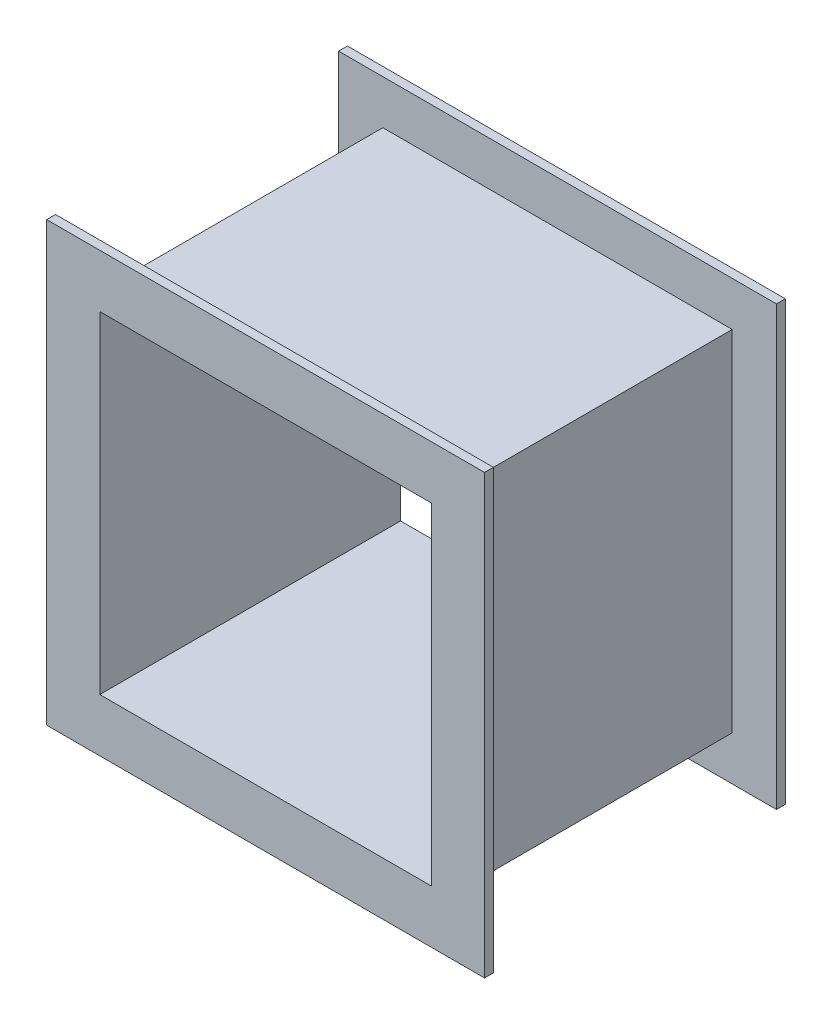
# Autodesk Inventor part: Измельчитель комков
Saved by Autodesk Inventor 2025 (Build 290162010, 162A)
## iProperties
Created: 2024-10-30
Part Number: Измельчитель комков
Material: Generic
Document SubType Name: Modeling
Designer: pokla
Density: 1 g/cm^3
Appearance: Default
Author: pokla
Autodesk Inventor part; units mm, degrees
ref_plane "YZ Plane" through (0, 0, 0) normal (1, 0, 0) x (0, 1, 0)
ref_plane "XZ Plane" through (0, 0, 0) normal (0, 1, 0) x (-1, 0, 0)
ref_plane "XY Plane" through (0, 0, 0) normal (0, 0, 1) x (1, 0, 0)
sketch "Sketch1" plane through (0, 0, 0) normal (0, 0, 1) x (1, 0, 0)
  line L0 (-247.5, 247.5) -> (247.5, 247.5)
  line L1 (247.5, 247.5) -> (247.5, -247.5)
  line L2 (247.5, -247.5) -> (-247.5, -247.5)
  line L3 (-247.5, -247.5) -> (-247.5, 247.5)
  line L4 (-247.5, -247.5) -> (247.5, 247.5) construction
  point P0 (0, 0)
  point P1 (0, 0)
  dimension "d0" = 495
  dimension "d1" = 495
  constraints: 10 end point, 2 parallel, 1 coincident, 1 horizontal, 1 midpoint, 1 perpendicular
  measures "d0" distance of L0.start L0.end
  measures "d1" distance of L2.end L0.start
extrude "Extrusion1" add sketch "Sketch1" against normal blind 10
sketch "Sketch2" plane through (0, 0, -10) normal (0, 0, -1) x (-1, 0, 0)
  line L0 (197.5, -197.5) -> (-197.5, -197.5)
  line L1 (-197.5, -197.5) -> (-197.5, 197.5)
  line L2 (-197.5, 197.5) -> (197.5, 197.5)
  line L3 (197.5, 197.5) -> (197.5, -197.5)
  line L4 (197.5, -197.5) -> (-197.5, 197.5) construction
  point P0 (0, 0)
  point P1 (0, 0)
  dimension "d4" = 395
  dimension "d5" = 395
  constraints: 10 end point, 2 parallel, 1 coincident, 1 horizontal, 1 midpoint, 1 perpendicular
  measures "d4" distance of L0.start L0.end
  measures "d5" distance of L2.end L0.start
extrude "Extrusion2" add sketch "Sketch2" along normal blind 320
sketch "Sketch3" plane through (0, 0, -330) normal (0, 0, -1) x (-1, 0, 0)
  line L0 (-247.5, -247.5) -> (247.5, -247.5)
  line L1 (247.5, -247.5) -> (247.5, 247.5)
  line L2 (247.5, 247.5) -> (-247.5, 247.5)
  line L3 (-247.5, 247.5) -> (-247.5, -247.5)
  line L4 (-247.5, -247.5) -> (247.5, 247.5) construction
  point P0 (0, 0)
  point P1 (0, 0)
  dimension "d8" = 495
  dimension "d9" = 495
  constraints: 10 end point, 2 parallel, 1 coincident, 1 horizontal, 1 midpoint, 1 perpendicular
  measures "d8" distance of L2.end L0.start
  measures "d9" distance of L0.start L0.end
extrude "Extrusion3" add sketch "Sketch3" along normal blind 10
sketch "Sketch4" plane through (0, 0, 0) normal (0, 0, 1) x (1, 0, 0)
  line L0 (-187.5, -187.5) -> (187.5, -187.5)
  line L1 (187.5, -187.5) -> (187.5, 187.5)
  line L2 (187.5, 187.5) -> (-187.5, 187.5)
  line L3 (-187.5, 187.5) -> (-187.5, -187.5)
  line L4 (-187.5, -187.5) -> (187.5, 187.5) construction
  point P0 (0, 0)
  point P1 (0, 0)
  dimension "d12" = 375
  dimension "d13" = 375
  constraints: 10 end point, 2 parallel, 1 coincident, 1 horizontal, 1 midpoint, 1 perpendicular
  measures "d12" distance of L2.end L0.start
  measures "d13" distance of L0.start L0.end
extrude "Extrusion4" cut sketch "Sketch4" against normal through all
equation "\"d1\" = d0"
equation "\"d5\" = d4"
equation "\"d8\" = d0"
equation "\"d9\" = d8"
body "Solid1"
